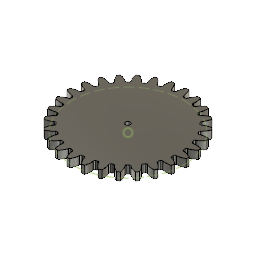
big_gear v6 (Autodesk Fusion 360 design; units mm, degrees)
description: Spur Gear; Module: 3.0; Num Teeth: 28; Pressure Angle: 20.0; Backlash: 0.00 mm
Autodesk Fusion 360 part; units mm, degrees
(part 1 of 4)
sketch "Sketch1" plane through (0, 0, 5) normal (0, 0, 1) x (-1, 0, 0)
  arc A0 (-25.3771, 2.9606) -> (-25.3996, 2.7606) centre (0, 0) ccw
  spline S0 degree 3 poles (-26.3672, 1.869) (-26.2575, 1.8719) (-26.149, 1.8929) (-25.9431, 1.9692) (-25.8472, 2.0241) (-25.6612, 2.1757) (-25.5772, 2.2768) (-25.4529, 2.5057) (-25.4137, 2.6311) (-25.3996, 2.7606) knots -0.143992 -0.143992 -0.143992 -0.143992 -0.11106 -0.11106 -0.078129 -0.078129 -0.039064 -0.039064 0 0 0 0
  spline S1 degree 3 poles (-29.9911, 0.731) (-29.3159, 1.0797) (-27.9521, 1.7065) (-26.5825, 1.8547) (-26.4748, 1.8661) (-26.3672, 1.869) knots -0.425485 -0.425485 -0.425485 -0.425485 -0.0445 -0.0445 -0.012227 -0.012227 -0.012227 -0.012227
  arc A1 (-29.9911, 0.731) -> (-29.9911, -0.731) centre (0, 0) ccw
  spline S2 degree 3 poles (-26.3672, -1.869) (-26.7354, -1.8592) (-27.3741, -1.7595) (-28.77, -1.3092) (-29.3991, -1.0367) (-29.9911, -0.731) knots -0.43899 -0.43899 -0.43899 -0.43899 -0.19989 -0.19989 0 0 0 0
  spline S3 degree 3 poles (-25.3996, -2.7606) (-25.4115, -2.6515) (-25.4412, -2.545) (-25.5341, -2.3461) (-25.5966, -2.255) (-25.7629, -2.0819) (-25.8706, -2.0065) (-26.1088, -1.9013) (-26.2371, -1.8725) (-26.3672, -1.869) knots -0.143992 -0.143992 -0.143992 -0.143992 -0.11106 -0.11106 -0.078129 -0.078129 -0.039064 -0.039064 0 0 0 0
  arc A2 (-25.3996, -2.7606) -> (-25.3771, -2.9606) centre (0, 0) ccw
  spline S4 degree 3 poles (-26.122, -4.0451) (-26.0157, -4.0179) (-25.9146, -3.9733) (-25.7309, -3.8531) (-25.6496, -3.7782) (-25.5019, -3.589) (-25.4426, -3.4717) (-25.3723, -3.221) (-25.362, -3.0899) (-25.3771, -2.9606) knots -0.143992 -0.143992 -0.143992 -0.143992 -0.11106 -0.11106 -0.078129 -0.078129 -0.039064 -0.039064 0 0 0 0
  spline S5 degree 3 poles (-29.4018, -5.961) (-28.8212, -5.4708) (-27.631, -4.5562) (-26.3288, -4.1069) (-26.2263, -4.0718) (-26.122, -4.0451) knots -0.425485 -0.425485 -0.425485 -0.425485 -0.0445 -0.0445 -0.012227 -0.012227 -0.012227 -0.012227
  arc A3 (-29.4018, -5.961) -> (-29.0765, -7.3863) centre (0, 0) ccw
  spline S6 degree 3 poles (-25.2903, -7.6894) (-25.6513, -7.7618) (-26.2963, -7.8067) (-27.7573, -7.6783) (-28.4313, -7.5527) (-29.0765, -7.3863) knots -0.43899 -0.43899 -0.43899 -0.43899 -0.19989 -0.19989 0 0 0 0
  spline S7 degree 3 poles (-24.1485, -8.3433) (-24.1844, -8.2396) (-24.237, -8.1424) (-24.3719, -7.9692) (-24.4531, -7.8942) (-24.6537, -7.7625) (-24.7755, -7.713) (-25.0311, -7.6634) (-25.1626, -7.6638) (-25.2903, -7.6894) knots -0.143992 -0.143992 -0.143992 -0.143992 -0.11106 -0.11106 -0.078129 -0.078129 -0.039064 -0.039064 0 0 0 0
  arc A4 (-24.1485, -8.3433) -> (-24.082, -8.5333) centre (0, 0) ccw
  spline S8 degree 3 poles (-24.567, -9.7564) (-24.4694, -9.7062) (-24.3807, -9.6402) (-24.2284, -9.4821) (-24.1657, -9.3911) (-24.0639, -9.1738) (-24.0322, -9.0462) (-24.0195, -8.7861) (-24.0386, -8.656) (-24.082, -8.5333) knots -0.143992 -0.143992 -0.143992 -0.143992 -0.11106 -0.11106 -0.078129 -0.078129 -0.039064 -0.039064 0 0 0 0
  spline S9 degree 3 poles (-27.3382, -12.3541) (-26.8812, -11.7469) (-25.9244, -10.5904) (-24.7548, -9.8627) (-24.6626, -9.8056) (-24.567, -9.7564) knots -0.425485 -0.425485 -0.425485 -0.425485 -0.0445 -0.0445 -0.012227 -0.012227 -0.012227 -0.012227
  arc A5 (-27.3382, -12.3541) -> (-26.7039, -13.6712) centre (0, 0) ccw
  spline S10 degree 3 poles (-22.9451, -13.1242) (-23.281, -13.2751) (-23.8998, -13.4625) (-25.3528, -13.6624) (-26.0379, -13.6899) (-26.7039, -13.6712) knots -0.43899 -0.43899 -0.43899 -0.43899 -0.19989 -0.19989 0 0 0 0
  spline S11 degree 3 poles (-21.6865, -13.5077) (-21.7445, -13.4145) (-21.8175, -13.3315) (-21.9875, -13.1926) (-22.0834, -13.1376) (-22.3083, -13.0538) (-22.438, -13.0327) (-22.6983, -13.0412) (-22.8263, -13.0709) (-22.9451, -13.1242) knots -0.143992 -0.143992 -0.143992 -0.143992 -0.11106 -0.11106 -0.078129 -0.078129 -0.039064 -0.039064 0 0 0 0
  arc A6 (-21.6865, -13.5077) -> (-21.5794, -13.6781) centre (0, 0) ccw
  spline S12 degree 3 poles (-21.78, -14.9785) (-21.6961, -14.9078) (-21.6243, -14.8237) (-21.5109, -14.6357) (-21.4701, -14.533) (-21.4192, -14.2985) (-21.4167, -14.167) (-21.4622, -13.9106) (-21.5097, -13.7881) (-21.5794, -13.6781) knots -0.143992 -0.143992 -0.143992 -0.143992 -0.11106 -0.11106 -0.078129 -0.078129 -0.039064 -0.039064 0 0 0 0
  spline S13 degree 3 poles (-23.9037, -18.1277) (-23.5933, -17.434) (-22.9178, -16.0936) (-21.9395, -15.1238) (-21.8623, -15.0477) (-21.78, -14.9785) knots -0.425485 -0.425485 -0.425485 -0.425485 -0.0445 -0.0445 -0.012227 -0.012227 -0.012227 -0.012227
  arc A7 (-23.9037, -18.1277) -> (-22.9922, -19.2706) centre (0, 0) ccw
  spline S14 degree 3 poles (-19.4494, -17.9009) (-19.7433, -18.1228) (-20.3049, -18.4432) (-21.677, -18.9614) (-22.3388, -19.1406) (-22.9922, -19.2706) knots -0.43899 -0.43899 -0.43899 -0.43899 -0.19989 -0.19989 0 0 0 0
  spline S15 degree 3 poles (-18.137, -17.9947) (-18.2143, -17.9168) (-18.304, -17.8521) (-18.5006, -17.7545) (-18.6063, -17.7222) (-18.8442, -17.6906) (-18.9754, -17.6988) (-19.2272, -17.7651) (-19.3455, -17.8225) (-19.4494, -17.9009) knots -0.143992 -0.143992 -0.143992 -0.143992 -0.11106 -0.11106 -0.078129 -0.078129 -0.039064 -0.039064 0 0 0 0
  arc A8 (-18.137, -17.9947) -> (-17.9947, -18.137) centre (0, 0) ccw
  spline S16 degree 3 poles (-17.9009, -19.4494) (-17.8348, -19.3618) (-17.7835, -19.2639) (-17.7149, -19.0554) (-17.6979, -18.9462) (-17.7005, -18.7062) (-17.7273, -18.5775) (-17.8286, -18.3376) (-17.9023, -18.2287) (-17.9947, -18.137) knots -0.143992 -0.143992 -0.143992 -0.143992 -0.11106 -0.11106 -0.078129 -0.078129 -0.039064 -0.039064 0 0 0 0
  spline S17 degree 3 poles (-19.2706, -22.9922) (-19.1223, -22.2469) (-18.762, -20.7898) (-18.024, -19.6266) (-17.9658, -19.5353) (-17.9009, -19.4494) knots -0.425485 -0.425485 -0.425485 -0.425485 -0.0445 -0.0445 -0.012227 -0.012227 -0.012227 -0.012227
  arc A9 (-19.2706, -22.9922) -> (-18.1277, -23.9037) centre (0, 0) ccw
  spline S18 degree 3 poles (-14.9785, -21.78) (-15.2156, -22.0617) (-15.6918, -22.499) (-16.9142, -23.3096) (-17.5195, -23.6315) (-18.1277, -23.9037) knots -0.43899 -0.43899 -0.43899 -0.43899 -0.19989 -0.19989 0 0 0 0
  spline S19 degree 3 poles (-13.6781, -21.5794) (-13.7708, -21.5207) (-13.8726, -21.4776) (-14.086, -21.4261) (-14.1962, -21.4182) (-14.4352, -21.4403) (-14.5613, -21.4775) (-14.7921, -21.5981) (-14.8946, -21.6804) (-14.9785, -21.78) knots -0.143992 -0.143992 -0.143992 -0.143992 -0.11106 -0.11106 -0.078129 -0.078129 -0.039064 -0.039064 0 0 0 0
  arc A10 (-13.6781, -21.5794) -> (-13.5077, -21.6865) centre (0, 0) ccw
  spline S20 degree 3 poles (-13.1242, -22.9451) (-13.0792, -22.845) (-13.051, -22.7381) (-13.0305, -22.5196) (-13.0383, -22.4093) (-13.0942, -22.1759) (-13.1489, -22.0564) (-13.3011, -21.8451) (-13.3972, -21.7553) (-13.5077, -21.6865) knots -0.143992 -0.143992 -0.143992 -0.143992 -0.11106 -0.11106 -0.078129 -0.078129 -0.039064 -0.039064 0 0 0 0
  spline S21 degree 3 poles (-13.6712, -26.7039) (-13.6925, -25.9443) (-13.6655, -24.4435) (-13.2048, -23.1453) (-13.1683, -23.0433) (-13.1242, -22.9451) knots -0.425485 -0.425485 -0.425485 -0.425485 -0.0445 -0.0445 -0.012227 -0.012227 -0.012227 -0.012227
  arc A11 (-13.6712, -26.7039) -> (-12.3541, -27.3382) centre (0, 0) ccw
  spline S22 degree 3 poles (-9.7564, -24.567) (-9.9249, -24.8944) (-10.2919, -25.4267) (-11.3032, -26.4889) (-11.8217, -26.9375) (-12.3541, -27.3382) knots -0.43899 -0.43899 -0.43899 -0.43899 -0.19989 -0.19989 0 0 0 0
  spline S23 degree 3 poles (-8.5333, -24.082) (-8.6367, -24.0454) (-8.7455, -24.026) (-8.9651, -24.0234) (-9.0743, -24.0401) (-9.3024, -24.1149) (-9.417, -24.1792) (-9.6152, -24.3482) (-9.6968, -24.4512) (-9.7564, -24.567) knots -0.143992 -0.143992 -0.143992 -0.143992 -0.11106 -0.11106 -0.078129 -0.078129 -0.039064 -0.039064 0 0 0 0
  arc A12 (-8.5333, -24.082) -> (-8.3433, -24.1485) centre (0, 0) ccw
  spline S24 degree 3 poles (-7.6894, -25.2903) (-7.6678, -25.1826) (-7.6641, -25.0722) (-7.6927, -24.8545) (-7.7249, -24.7488) (-7.8313, -24.5336) (-7.9112, -24.4293) (-8.1067, -24.2572) (-8.2203, -24.191) (-8.3433, -24.1485) knots -0.143992 -0.143992 -0.143992 -0.143992 -0.11106 -0.11106 -0.078129 -0.078129 -0.039064 -0.039064 0 0 0 0
  spline S25 degree 3 poles (-7.3863, -29.0765) (-7.576, -28.3406) (-7.8837, -26.8715) (-7.7234, -25.5033) (-7.7105, -25.3957) (-7.6894, -25.2903) knots -0.425485 -0.425485 -0.425485 -0.425485 -0.0445 -0.0445 -0.012227 -0.012227 -0.012227 -0.012227
  arc A13 (-7.3863, -29.0765) -> (-5.961, -29.4018) centre (0, 0) ccw
  spline S26 degree 3 poles (-4.0451, -26.122) (-4.1366, -26.4788) (-4.3759, -27.0793) (-5.1255, -28.34) (-5.5312, -28.8927) (-5.961, -29.4018) knots -0.43899 -0.43899 -0.43899 -0.43899 -0.19989 -0.19989 0 0 0 0
  spline S27 degree 3 poles (-2.9606, -25.3771) (-3.0696, -25.3644) (-3.18, -25.3697) (-3.3946, -25.416) (-3.4974, -25.4566) (-3.7031, -25.5802) (-3.8005, -25.6685) (-3.9561, -25.8773) (-4.0128, -25.9959) (-4.0451, -26.122) knots -0.143992 -0.143992 -0.143992 -0.143992 -0.11106 -0.11106 -0.078129 -0.078129 -0.039064 -0.039064 0 0 0 0
  arc A14 (-2.9606, -25.3771) -> (-2.7606, -25.3996) centre (0, 0) ccw
  spline S28 degree 3 poles (-1.869, -26.3672) (-1.8719, -26.2575) (-1.8929, -26.149) (-1.9692, -25.9431) (-2.0241, -25.8472) (-2.1757, -25.6612) (-2.2768, -25.5772) (-2.5057, -25.4529) (-2.6311, -25.4137) (-2.7606, -25.3996) knots -0.143992 -0.143992 -0.143992 -0.143992 -0.11106 -0.11106 -0.078129 -0.078129 -0.039064 -0.039064 0 0 0 0
  spline S29 degree 3 poles (-0.731, -29.9911) (-1.0797, -29.3159) (-1.7065, -27.9521) (-1.8547, -26.5825) (-1.8661, -26.4748) (-1.869, -26.3672) knots -0.425485 -0.425485 -0.425485 -0.425485 -0.0445 -0.0445 -0.012227 -0.012227 -0.012227 -0.012227
  arc A15 (-0.731, -29.9911) -> (0.731, -29.9911) centre (0, 0) ccw
  spline S30 degree 3 poles (1.869, -26.3672) (1.8592, -26.7354) (1.7595, -27.3741) (1.3092, -28.77) (1.0367, -29.3991) (0.731, -29.9911) knots -0.43899 -0.43899 -0.43899 -0.43899 -0.19989 -0.19989 0 0 0 0
  spline S31 degree 3 poles (2.7606, -25.3996) (2.6515, -25.4115) (2.545, -25.4412) (2.3461, -25.5341) (2.255, -25.5966) (2.0819, -25.7629) (2.0065, -25.8706) (1.9013, -26.1088) (1.8725, -26.2371) (1.869, -26.3672) knots -0.143992 -0.143992 -0.143992 -0.143992 -0.11106 -0.11106 -0.078129 -0.078129 -0.039064 -0.039064 0 0 0 0
  arc A16 (2.7606, -25.3996) -> (2.9606, -25.3771) centre (0, 0) ccw
  spline S32 degree 3 poles (4.0451, -26.122) (4.0179, -26.0157) (3.9733, -25.9146) (3.8531, -25.7309) (3.7782, -25.6496) (3.589, -25.5019) (3.4717, -25.4426) (3.221, -25.3723) (3.0899, -25.362) (2.9606, -25.3771) knots -0.143992 -0.143992 -0.143992 -0.143992 -0.11106 -0.11106 -0.078129 -0.078129 -0.039064 -0.039064 0 0 0 0
  spline S33 degree 3 poles (5.961, -29.4018) (5.4708, -28.8212) (4.5562, -27.631) (4.1069, -26.3288) (4.0718, -26.2263) (4.0451, -26.122) knots -0.425485 -0.425485 -0.425485 -0.425485 -0.0445 -0.0445 -0.012227 -0.012227 -0.012227 -0.012227
  arc A17 (5.961, -29.4018) -> (7.3863, -29.0765) centre (0, 0) ccw
  spline S34 degree 3 poles (7.6894, -25.2903) (7.7618, -25.6513) (7.8067, -26.2963) (7.6783, -27.7573) (7.5527, -28.4313) (7.3863, -29.0765) knots -0.43899 -0.43899 -0.43899 -0.43899 -0.19989 -0.19989 0 0 0 0
  spline S35 degree 3 poles (8.3433, -24.1485) (8.2396, -24.1844) (8.1424, -24.237) (7.9692, -24.3719) (7.8942, -24.4531) (7.7625, -24.6537) (7.713, -24.7755) (7.6634, -25.0311) (7.6638, -25.1626) (7.6894, -25.2903) knots -0.143992 -0.143992 -0.143992 -0.143992 -0.11106 -0.11106 -0.078129 -0.078129 -0.039064 -0.039064 0 0 0 0
  arc A18 (8.3433, -24.1485) -> (8.5333, -24.082) centre (0, 0) ccw
  spline S36 degree 3 poles (9.7564, -24.567) (9.7062, -24.4694) (9.6402, -24.3807) (9.4821, -24.2284) (9.3911, -24.1657) (9.1738, -24.0639) (9.0462, -24.0322) (8.7861, -24.0195) (8.656, -24.0386) (8.5333, -24.082) knots -0.143992 -0.143992 -0.143992 -0.143992 -0.11106 -0.11106 -0.078129 -0.078129 -0.039064 -0.039064 0 0 0 0
  spline S37 degree 3 poles (12.3541, -27.3382) (11.7469, -26.8812) (10.5904, -25.9244) (9.8627, -24.7548) (9.8056, -24.6626) (9.7564, -24.567) knots -0.425485 -0.425485 -0.425485 -0.425485 -0.0445 -0.0445 -0.012227 -0.012227 -0.012227 -0.012227
  arc A19 (12.3541, -27.3382) -> (13.6712, -26.7039) centre (0, 0) ccw
  spline S38 degree 3 poles (13.1242, -22.9451) (13.2751, -23.281) (13.4625, -23.8998) (13.6624, -25.3528) (13.6899, -26.0379) (13.6712, -26.7039) knots -0.43899 -0.43899 -0.43899 -0.43899 -0.19989 -0.19989 0 0 0 0
  spline S39 degree 3 poles (13.5077, -21.6865) (13.4145, -21.7445) (13.3315, -21.8175) (13.1926, -21.9875) (13.1376, -22.0834) (13.0538, -22.3083) (13.0327, -22.438) (13.0412, -22.6983) (13.0709, -22.8263) (13.1242, -22.9451) knots -0.143992 -0.143992 -0.143992 -0.143992 -0.11106 -0.11106 -0.078129 -0.078129 -0.039064 -0.039064 0 0 0 0
  arc A20 (13.5077, -21.6865) -> (13.6781, -21.5794) centre (0, 0) ccw
  spline S40 degree 3 poles (14.9785, -21.78) (14.9078, -21.6961) (14.8237, -21.6243) (14.6357, -21.5109) (14.533, -21.4701) (14.2985, -21.4192) (14.167, -21.4167) (13.9106, -21.4622) (13.7881, -21.5097) (13.6781, -21.5794) knots -0.143992 -0.143992 -0.143992 -0.143992 -0.11106 -0.11106 -0.078129 -0.078129 -0.039064 -0.039064 0 0 0 0
  spline S41 degree 3 poles (18.1277, -23.9037) (17.434, -23.5933) (16.0936, -22.9178) (15.1238, -21.9395) (15.0477, -21.8623) (14.9785, -21.78) knots -0.425485 -0.425485 -0.425485 -0.425485 -0.0445 -0.0445 -0.012227 -0.012227 -0.012227 -0.012227
  arc A21 (18.1277, -23.9037) -> (19.2706, -22.9922) centre (0, 0) ccw
  spline S42 degree 3 poles (17.9009, -19.4494) (18.1228, -19.7433) (18.4432, -20.3049) (18.9614, -21.677) (19.1406, -22.3388) (19.2706, -22.9922) knots -0.43899 -0.43899 -0.43899 -0.43899 -0.19989 -0.19989 0 0 0 0
  spline S43 degree 3 poles (17.9947, -18.137) (17.9168, -18.2143) (17.8521, -18.304) (17.7545, -18.5006) (17.7222, -18.6063) (17.6906, -18.8442) (17.6988, -18.9754) (17.7651, -19.2272) (17.8225, -19.3455) (17.9009, -19.4494) knots -0.143992 -0.143992 -0.143992 -0.143992 -0.11106 -0.11106 -0.078129 -0.078129 -0.039064 -0.039064 0 0 0 0
  arc A22 (17.9947, -18.137) -> (18.137, -17.9947) centre (0, 0) ccw
  spline S44 degree 3 poles (19.4494, -17.9009) (19.3618, -17.8348) (19.2639, -17.7835) (19.0554, -17.7149) (18.9462, -17.6979) (18.7062, -17.7005) (18.5775, -17.7273) (18.3376, -17.8286) (18.2287, -17.9023) (18.137, -17.9947) knots -0.143992 -0.143992 -0.143992 -0.143992 -0.11106 -0.11106 -0.078129 -0.078129 -0.039064 -0.039064 0 0 0 0
  spline S45 degree 3 poles (22.9922, -19.2706) (22.2469, -19.1223) (20.7898, -18.762) (19.6266, -18.024) (19.5353, -17.9658) (19.4494, -17.9009) knots -0.425485 -0.425485 -0.425485 -0.425485 -0.0445 -0.0445 -0.012227 -0.012227 -0.012227 -0.012227
  arc A23 (22.9922, -19.2706) -> (23.9037, -18.1277) centre (0, 0) ccw
  spline S46 degree 3 poles (21.78, -14.9785) (22.0617, -15.2156) (22.499, -15.6918) (23.3096, -16.9142) (23.6315, -17.5195) (23.9037, -18.1277) knots -0.43899 -0.43899 -0.43899 -0.43899 -0.19989 -0.19989 0 0 0 0
  spline S47 degree 3 poles (21.5794, -13.6781) (21.5207, -13.7708) (21.4776, -13.8726) (21.4261, -14.086) (21.4182, -14.1962) (21.4403, -14.4352) (21.4775, -14.5613) (21.5981, -14.7921) (21.6804, -14.8946) (21.78, -14.9785) knots -0.143992 -0.143992 -0.143992 -0.143992 -0.11106 -0.11106 -0.078129 -0.078129 -0.039064 -0.039064 0 0 0 0
  arc A24 (21.5794, -13.6781) -> (21.6865, -13.5077) centre (0, 0) ccw
  spline S48 degree 3 poles (22.9451, -13.1242) (22.845, -13.0792) (22.7381, -13.051) (22.5196, -13.0305) (22.4093, -13.0383) (22.1759, -13.0942) (22.0564, -13.1489) (21.8451, -13.3011) (21.7553, -13.3972) (21.6865, -13.5077) knots -0.143992 -0.143992 -0.143992 -0.143992 -0.11106 -0.11106 -0.078129 -0.078129 -0.039064 -0.039064 0 0 0 0
  spline S49 degree 3 poles (26.7039, -13.6712) (25.9443, -13.6925) (24.4435, -13.6655) (23.1453, -13.2048) (23.0433, -13.1683) (22.9451, -13.1242) knots -0.425485 -0.425485 -0.425485 -0.425485 -0.0445 -0.0445 -0.012227 -0.012227 -0.012227 -0.012227
  arc A25 (26.7039, -13.6712) -> (27.3382, -12.3541) centre (0, 0) ccw
  spline S50 degree 3 poles (24.567, -9.7564) (24.8944, -9.9249) (25.4267, -10.2919) (26.4889, -11.3032) (26.9375, -11.8217) (27.3382, -12.3541) knots -0.43899 -0.43899 -0.43899 -0.43899 -0.19989 -0.19989 0 0 0 0
  spline S51 degree 3 poles (24.082, -8.5333) (24.0454, -8.6367) (24.026, -8.7455) (24.0234, -8.9651) (24.0401, -9.0743) (24.1149, -9.3024) (24.1792, -9.417) (24.3482, -9.6152) (24.4512, -9.6968) (24.567, -9.7564) knots -0.143992 -0.143992 -0.143992 -0.143992 -0.11106 -0.11106 -0.078129 -0.078129 -0.039064 -0.039064 0 0 0 0
  arc A26 (24.082, -8.5333) -> (24.1485, -8.3433) centre (0, 0) ccw
  spline S52 degree 3 poles (25.2903, -7.6894) (25.1826, -7.6678) (25.0722, -7.6641) (24.8545, -7.6927) (24.7488, -7.7249) (24.5336, -7.8313) (24.4293, -7.9112) (24.2572, -8.1067) (24.191, -8.2203) (24.1485, -8.3433) knots -0.143992 -0.143992 -0.143992 -0.143992 -0.11106 -0.11106 -0.078129 -0.078129 -0.039064 -0.039064 0 0 0 0
  spline S53 degree 3 poles (29.0765, -7.3863) (28.3406, -7.576) (26.8715, -7.8837) (25.5033, -7.7234) (25.3957, -7.7105) (25.2903, -7.6894) knots -0.425485 -0.425485 -0.425485 -0.425485 -0.0445 -0.0445 -0.012227 -0.012227 -0.012227 -0.012227
  arc A27 (29.0765, -7.3863) -> (29.4018, -5.961) centre (0, 0) ccw
  spline S54 degree 3 poles (26.122, -4.0451) (26.4788, -4.1366) (27.0793, -4.3759) (28.34, -5.1255) (28.8927, -5.5312) (29.4018, -5.961) knots -0.43899 -0.43899 -0.43899 -0.43899 -0.19989 -0.19989 0 0 0 0
  spline S55 degree 3 poles (25.3771, -2.9606) (25.3644, -3.0696) (25.3697, -3.18) (25.416, -3.3946) (25.4566, -3.4974) (25.5802, -3.7031) (25.6685, -3.8005) (25.8773, -3.9561) (25.9959, -4.0128) (26.122, -4.0451) knots -0.143992 -0.143992 -0.143992 -0.143992 -0.11106 -0.11106 -0.078129 -0.078129 -0.039064 -0.039064 0 0 0 0
  arc A28 (25.3771, -2.9606) -> (25.3996, -2.7606) centre (0, 0) ccw
  spline S56 degree 3 poles (26.3672, -1.869) (26.2575, -1.8719) (26.149, -1.8929) (25.9431, -1.9692) (25.8472, -2.0241) (25.6612, -2.1757) (25.5772, -2.2768) (25.4529, -2.5057) (25.4137, -2.6311) (25.3996, -2.7606) knots -0.143992 -0.143992 -0.143992 -0.143992 -0.11106 -0.11106 -0.078129 -0.078129 -0.039064 -0.039064 0 0 0 0
  spline S57 degree 3 poles (29.9911, -0.731) (29.3159, -1.0797) (27.9521, -1.7065) (26.5825, -1.8547) (26.4748, -1.8661) (26.3672, -1.869) knots -0.425485 -0.425485 -0.425485 -0.425485 -0.0445 -0.0445 -0.012227 -0.012227 -0.012227 -0.012227
  arc A29 (29.9911, -0.731) -> (29.9911, 0.731) centre (0, 0) ccw
  spline S58 degree 3 poles (26.3672, 1.869) (26.7354, 1.8592) (27.3741, 1.7595) (28.77, 1.3092) (29.3991, 1.0367) (29.9911, 0.731) knots -0.43899 -0.43899 -0.43899 -0.43899 -0.19989 -0.19989 0 0 0 0
  spline S59 degree 3 poles (25.3996, 2.7606) (25.4115, 2.6515) (25.4412, 2.545) (25.5341, 2.3461) (25.5966, 2.255) (25.7629, 2.0819) (25.8706, 2.0065) (26.1088, 1.9013) (26.2371, 1.8725) (26.3672, 1.869) knots -0.143992 -0.143992 -0.143992 -0.143992 -0.11106 -0.11106 -0.078129 -0.078129 -0.039064 -0.039064 0 0 0 0
  arc A30 (25.3996, 2.7606) -> (25.3771, 2.9606) centre (0, 0) ccw
  spline S60 degree 3 poles (26.122, 4.0451) (26.0157, 4.0179) (25.9146, 3.9733) (25.7309, 3.8531) (25.6496, 3.7782) (25.5019, 3.589) (25.4426, 3.4717) (25.3723, 3.221) (25.362, 3.0899) (25.3771, 2.9606) knots -0.143992 -0.143992 -0.143992 -0.143992 -0.11106 -0.11106 -0.078129 -0.078129 -0.039064 -0.039064 0 0 0 0
  spline S61 degree 3 poles (29.4018, 5.961) (28.8212, 5.4708) (27.631, 4.5562) (26.3288, 4.1069) (26.2263, 4.0718) (26.122, 4.0451) knots -0.425485 -0.425485 -0.425485 -0.425485 -0.0445 -0.0445 -0.012227 -0.012227 -0.012227 -0.012227
  arc A31 (29.4018, 5.961) -> (29.0765, 7.3863) centre (0, 0) ccw
  spline S62 degree 3 poles (25.2903, 7.6894) (25.6513, 7.7618) (26.2963, 7.8067) (27.7573, 7.6783) (28.4313, 7.5527) (29.0765, 7.3863) knots -0.43899 -0.43899 -0.43899 -0.43899 -0.19989 -0.19989 0 0 0 0
  spline S63 degree 3 poles (24.1485, 8.3433) (24.1844, 8.2396) (24.237, 8.1424) (24.3719, 7.9692) (24.4531, 7.8942) (24.6537, 7.7625) (24.7755, 7.713) (25.0311, 7.6634) (25.1626, 7.6638) (25.2903, 7.6894) knots -0.143992 -0.143992 -0.143992 -0.143992 -0.11106 -0.11106 -0.078129 -0.078129 -0.039064 -0.039064 0 0 0 0
  arc A32 (24.1485, 8.3433) -> (24.082, 8.5333) centre (0, 0) ccw
  spline S64 degree 3 poles (24.567, 9.7564) (24.4694, 9.7062) (24.3807, 9.6402) (24.2284, 9.4821) (24.1657, 9.3911) (24.0639, 9.1738) (24.0322, 9.0462) (24.0195, 8.7861) (24.0386, 8.656) (24.082, 8.5333) knots -0.143992 -0.143992 -0.143992 -0.143992 -0.11106 -0.11106 -0.078129 -0.078129 -0.039064 -0.039064 0 0 0 0
  spline S65 degree 3 poles (27.3382, 12.3541) (26.8812, 11.7469) (25.9244, 10.5904) (24.7548, 9.8627) (24.6626, 9.8056) (24.567, 9.7564) knots -0.425485 -0.425485 -0.425485 -0.425485 -0.0445 -0.0445 -0.012227 -0.012227 -0.012227 -0.012227
  arc A33 (27.3382, 12.3541) -> (26.7039, 13.6712) centre (0, 0) ccw
  spline S66 degree 3 poles (22.9451, 13.1242) (23.281, 13.2751) (23.8998, 13.4625) (25.3528, 13.6624) (26.0379, 13.6899) (26.7039, 13.6712) knots -0.43899 -0.43899 -0.43899 -0.43899 -0.19989 -0.19989 0 0 0 0
  spline S67 degree 3 poles (21.6865, 13.5077) (21.7445, 13.4145) (21.8175, 13.3315) (21.9875, 13.1926) (22.0834, 13.1376) (22.3083, 13.0538) (22.438, 13.0327) (22.6983, 13.0412) (22.8263, 13.0709) (22.9451, 13.1242) knots -0.143992 -0.143992 -0.143992 -0.143992 -0.11106 -0.11106 -0.078129 -0.078129 -0.039064 -0.039064 0 0 0 0
  arc A34 (21.6865, 13.5077) -> (21.5794, 13.6781) centre (0, 0) ccw
  spline S68 degree 3 poles (21.78, 14.9785) (21.6961, 14.9078) (21.6243, 14.8237) (21.5109, 14.6357) (21.4701, 14.533) (21.4192, 14.2985) (21.4167, 14.167) (21.4622, 13.9106) (21.5097, 13.7881) (21.5794, 13.6781) knots -0.143992 -0.143992 -0.143992 -0.143992 -0.11106 -0.11106 -0.078129 -0.078129 -0.039064 -0.039064 0 0 0 0
  spline S69 degree 3 poles (23.9037, 18.1277) (23.5933, 17.434) (22.9178, 16.0936) (21.9395, 15.1238) (21.8623, 15.0477) (21.78, 14.9785) knots -0.425485 -0.425485 -0.425485 -0.425485 -0.0445 -0.0445 -0.012227 -0.012227 -0.012227 -0.012227
  arc A35 (23.9037, 18.1277) -> (22.9922, 19.2706) centre (0, 0) ccw
  spline S70 degree 3 poles (19.4494, 17.9009) (19.7433, 18.1228) (20.3049, 18.4432) (21.677, 18.9614) (22.3388, 19.1406) (22.9922, 19.2706) knots -0.43899 -0.43899 -0.43899 -0.43899 -0.19989 -0.19989 0 0 0 0
  spline S71 degree 3 poles (18.137, 17.9947) (18.2143, 17.9168) (18.304, 17.8521) (18.5006, 17.7545) (18.6063, 17.7222) (18.8442, 17.6906) (18.9754, 17.6988) (19.2272, 17.7651) (19.3455, 17.8225) (19.4494, 17.9009) knots -0.143992 -0.143992 -0.143992 -0.143992 -0.11106 -0.11106 -0.078129 -0.078129 -0.039064 -0.039064 0 0 0 0
  arc A36 (18.137, 17.9947) -> (17.9947, 18.137) centre (0, 0) ccw
  spline S72 degree 3 poles (17.9009, 19.4494) (17.8348, 19.3618) (17.7835, 19.2639) (17.7149, 19.0554) (17.6979, 18.9462) (17.7005, 18.7062) (17.7273, 18.5775) (17.8286, 18.3376) (17.9023, 18.2287) (17.9947, 18.137) knots -0.143992 -0.143992 -0.143992 -0.143992 -0.11106 -0.11106 -0.078129 -0.078129 -0.039064 -0.039064 0 0 0 0
  spline S73 degree 3 poles (19.2706, 22.9922) (19.1223, 22.2469) (18.762, 20.7898) (18.024, 19.6266) (17.9658, 19.5353) (17.9009, 19.4494) knots -0.425485 -0.425485 -0.425485 -0.425485 -0.0445 -0.0445 -0.012227 -0.012227 -0.012227 -0.012227
  arc A37 (19.2706, 22.9922) -> (18.1277, 23.9037) centre (0, 0) ccw
  spline S74 degree 3 poles (14.9785, 21.78) (15.2156, 22.0617) (15.6918, 22.499) (16.9142, 23.3096) (17.5195, 23.6315) (18.1277, 23.9037) knots -0.43899 -0.43899 -0.43899 -0.43899 -0.19989 -0.19989 0 0 0 0
  spline S75 degree 3 poles (13.6781, 21.5794) (13.7708, 21.5207) (13.8726, 21.4776) (14.086, 21.4261) (14.1962, 21.4182) (14.4352, 21.4403) (14.5613, 21.4775) (14.7921, 21.5981) (14.8946, 21.6804) (14.9785, 21.78) knots -0.143992 -0.143992 -0.143992 -0.143992 -0.11106 -0.11106 -0.078129 -0.078129 -0.039064 -0.039064 0 0 0 0
  arc A38 (13.6781, 21.5794) -> (13.5077, 21.6865) centre (0, 0) ccw
  spline S76 degree 3 poles (13.1242, 22.9451) (13.0792, 22.845) (13.051, 22.7381) (13.0305, 22.5196) (13.0383, 22.4093) (13.0942, 22.1759) (13.1489, 22.0564) (13.3011, 21.8451) (13.3972, 21.7553) (13.5077, 21.6865) knots -0.143992 -0.143992 -0.143992 -0.143992 -0.11106 -0.11106 -0.078129 -0.078129 -0.039064 -0.039064 0 0 0 0
  spline S77 degree 3 poles (13.6712, 26.7039) (13.6925, 25.9443) (13.6655, 24.4435) (13.2048, 23.1453) (13.1683, 23.0433) (13.1242, 22.9451) knots -0.425485 -0.425485 -0.425485 -0.425485 -0.0445 -0.0445 -0.012227 -0.012227 -0.012227 -0.012227
  arc A39 (13.6712, 26.7039) -> (12.3541, 27.3382) centre (0, 0) ccw
  spline S78 degree 3 poles (9.7564, 24.567) (9.9249, 24.8944) (10.2919, 25.4267) (11.3032, 26.4889) (11.8217, 26.9375) (12.3541, 27.3382) knots -0.43899 -0.43899 -0.43899 -0.43899 -0.19989 -0.19989 0 0 0 0
  spline S79 degree 3 poles (8.5333, 24.082) (8.6367, 24.0454) (8.7455, 24.026) (8.9651, 24.0234) (9.0743, 24.0401) (9.3024, 24.1149) (9.417, 24.1792) (9.6152, 24.3482) (9.6968, 24.4512) (9.7564, 24.567) knots -0.143992 -0.143992 -0.143992 -0.143992 -0.11106 -0.11106 -0.078129 -0.078129 -0.039064 -0.039064 0 0 0 0
  arc A40 (8.5333, 24.082) -> (8.3433, 24.1485) centre (0, 0) ccw
  spline S80 degree 3 poles (7.6894, 25.2903) (7.6678, 25.1826) (7.6641, 25.0722) (7.6927, 24.8545) (7.7249, 24.7488) (7.8313, 24.5336) (7.9112, 24.4293) (8.1067, 24.2572) (8.2203, 24.191) (8.3433, 24.1485) knots -0.143992 -0.143992 -0.143992 -0.143992 -0.11106 -0.11106 -0.078129 -0.078129 -0.039064 -0.039064 0 0 0 0
  spline S81 degree 3 poles (7.3863, 29.0765) (7.576, 28.3406) (7.8837, 26.8715) (7.7234, 25.5033) (7.7105, 25.3957) (7.6894, 25.2903) knots -0.425485 -0.425485 -0.425485 -0.425485 -0.0445 -0.0445 -0.012227 -0.012227 -0.012227 -0.012227
  arc A41 (7.3863, 29.0765) -> (5.961, 29.4018) centre (0, 0) ccw
  spline S82 degree 3 poles (4.0451, 26.122) (4.1366, 26.4788) (4.3759, 27.0793) (5.1255, 28.34) (5.5312, 28.8927) (5.961, 29.4018) knots -0.43899 -0.43899 -0.43899 -0.43899 -0.19989 -0.19989 0 0 0 0
  spline S83 degree 3 poles (2.9606, 25.3771) (3.0696, 25.3644) (3.18, 25.3697) (3.3946, 25.416) (3.4974, 25.4566) (3.7031, 25.5802) (3.8005, 25.6685) (3.9561, 25.8773) (4.0128, 25.9959) (4.0451, 26.122) knots -0.143992 -0.143992 -0.143992 -0.143992 -0.11106 -0.11106 -0.078129 -0.078129 -0.039064 -0.039064 0 0 0 0
  arc A42 (2.9606, 25.3771) -> (2.7606, 25.3996) centre (0, 0) ccw
  spline S84 degree 3 poles (1.869, 26.3672) (1.8719, 26.2575) (1.8929, 26.149) (1.9692, 25.9431) (2.0241, 25.8472) (2.1757, 25.6612) (2.2768, 25.5772) (2.5057, 25.4529) (2.6311, 25.4137) (2.7606, 25.3996) knots -0.143992 -0.143992 -0.143992 -0.143992 -0.11106 -0.11106 -0.078129 -0.078129 -0.039064 -0.039064 0 0 0 0
  spline S85 degree 3 poles (0.731, 29.9911) (1.0797, 29.3159) (1.7065, 27.9521) (1.8547, 26.5825) (1.8661, 26.4748) (1.869, 26.3672) knots -0.425485 -0.425485 -0.425485 -0.425485 -0.0445 -0.0445 -0.012227 -0.012227 -0.012227 -0.012227
  arc A43 (0.731, 29.9911) -> (-0.731, 29.9911) centre (0, 0) ccw
  spline S86 degree 3 poles (-1.869, 26.3672) (-1.8592, 26.7354) (-1.7595, 27.3741) (-1.3092, 28.77) (-1.0367, 29.3991) (-0.731, 29.9911) knots -0.43899 -0.43899 -0.43899 -0.43899 -0.19989 -0.19989 0 0 0 0
  spline S87 degree 3 poles (-2.7606, 25.3996) (-2.6515, 25.4115) (-2.545, 25.4412) (-2.3461, 25.5341) (-2.255, 25.5966) (-2.0819, 25.7629) (-2.0065, 25.8706) (-1.9013, 26.1088) (-1.8725, 26.2371) (-1.869, 26.3672) knots -0.143992 -0.143992 -0.143992 -0.143992 -0.11106 -0.11106 -0.078129 -0.078129 -0.039064 -0.039064 0 0 0 0
  arc A44 (-2.7606, 25.3996) -> (-2.9606, 25.3771) centre (0, 0) ccw
  spline S88 degree 3 poles (-4.0451, 26.122) (-4.0179, 26.0157) (-3.9733, 25.9146) (-3.8531, 25.7309) (-3.7782, 25.6496) (-3.589, 25.5019) (-3.4717, 25.4426) (-3.221, 25.3723) (-3.0899, 25.362) (-2.9606, 25.3771) knots -0.143992 -0.143992 -0.143992 -0.143992 -0.11106 -0.11106 -0.078129 -0.078129 -0.039064 -0.039064 0 0 0 0
  spline S89 degree 3 poles (-5.961, 29.4018) (-5.4708, 28.8212) (-4.5562, 27.631) (-4.1069, 26.3288) (-4.0718, 26.2263) (-4.0451, 26.122) knots -0.425485 -0.425485 -0.425485 -0.425485 -0.0445 -0.0445 -0.012227 -0.012227 -0.012227 -0.012227
  arc A45 (-5.961, 29.4018) -> (-7.3863, 29.0765) centre (0, 0) ccw
  spline S90 degree 3 poles (-7.6894, 25.2903) (-7.7618, 25.6513) (-7.8067, 26.2963) (-7.6783, 27.7573) (-7.5527, 28.4313) (-7.3863, 29.0765) knots -0.43899 -0.43899 -0.43899 -0.43899 -0.19989 -0.19989 0 0 0 0
  spline S91 degree 3 poles (-8.3433, 24.1485) (-8.2396, 24.1844) (-8.1424, 24.237) (-7.9692, 24.3719) (-7.8942, 24.4531) (-7.7625, 24.6537) (-7.713, 24.7755) (-7.6634, 25.0311) (-7.6638, 25.1626) (-7.6894, 25.2903) knots -0.143992 -0.143992 -0.143992 -0.143992 -0.11106 -0.11106 -0.078129 -0.078129 -0.039064 -0.039064 0 0 0 0
  arc A46 (-8.3433, 24.1485) -> (-8.5333, 24.082) centre (0, 0) ccw
  spline S92 degree 3 poles (-9.7564, 24.567) (-9.7062, 24.4694) (-9.6402, 24.3807) (-9.4821, 24.2284) (-9.3911, 24.1657) (-9.1738, 24.0639) (-9.0462, 24.0322) (-8.7861, 24.0195) (-8.656, 24.0386) (-8.5333, 24.082) knots -0.143992 -0.143992 -0.143992 -0.143992 -0.11106 -0.11106 -0.078129 -0.078129 -0.039064 -0.039064 0 0 0 0
  spline S93 degree 3 poles (-12.3541, 27.3382) (-11.7469, 26.8812) (-10.5904, 25.9244) (-9.8627, 24.7548) (-9.8056, 24.6626) (-9.7564, 24.567) knots -0.425485 -0.425485 -0.425485 -0.425485 -0.0445 -0.0445 -0.012227 -0.012227 -0.012227 -0.012227
  arc A47 (-12.3541, 27.3382) -> (-13.6712, 26.7039) centre (0, 0) ccw
  spline S94 degree 3 poles (-13.1242, 22.9451) (-13.2751, 23.281) (-13.4625, 23.8998) (-13.6624, 25.3528) (-13.6899, 26.0379) (-13.6712, 26.7039) knots -0.43899 -0.43899 -0.43899 -0.43899 -0.19989 -0.19989 0 0 0 0
  spline S95 degree 3 poles (-13.5077, 21.6865) (-13.4145, 21.7445) (-13.3315, 21.8175) (-13.1926, 21.9875) (-13.1376, 22.0834) (-13.0538, 22.3083) (-13.0327, 22.438) (-13.0412, 22.6983) (-13.0709, 22.8263) (-13.1242, 22.9451) knots -0.143992 -0.143992 -0.143992 -0.143992 -0.11106 -0.11106 -0.078129 -0.078129 -0.039064 -0.039064 0 0 0 0
  arc A48 (-13.5077, 21.6865) -> (-13.6781, 21.5794) centre (0, 0) ccw
  spline S96 degree 3 poles (-14.9785, 21.78) (-14.9078, 21.6961) (-14.8237, 21.6243) (-14.6357, 21.5109) (-14.533, 21.4701) (-14.2985, 21.4192) (-14.167, 21.4167) (-13.9106, 21.4622) (-13.7881, 21.5097) (-13.6781, 21.5794) knots -0.143992 -0.143992 -0.143992 -0.143992 -0.11106 -0.11106 -0.078129 -0.078129 -0.039064 -0.039064 0 0 0 0
  spline S97 degree 3 poles (-18.1277, 23.9037) (-17.434, 23.5933) (-16.0936, 22.9178) (-15.1238, 21.9395) (-15.0477, 21.8623) (-14.9785, 21.78) knots -0.425485 -0.425485 -0.425485 -0.425485 -0.0445 -0.0445 -0.012227 -0.012227 -0.012227 -0.012227
  arc A49 (-18.1277, 23.9037) -> (-19.2706, 22.9922) centre (0, 0) ccw
  spline S98 degree 3 poles (-17.9009, 19.4494) (-18.1228, 19.7433) (-18.4432, 20.3049) (-18.9614, 21.677) (-19.1406, 22.3388) (-19.2706, 22.9922) knots -0.43899 -0.43899 -0.43899 -0.43899 -0.19989 -0.19989 0 0 0 0
  spline S99 degree 3 poles (-17.9947, 18.137) (-17.9168, 18.2143) (-17.8521, 18.304) (-17.7545, 18.5006) (-17.7222, 18.6063) (-17.6906, 18.8442) (-17.6988, 18.9754) (-17.7651, 19.2272) (-17.8225, 19.3455) (-17.9009, 19.4494) knots -0.143992 -0.143992 -0.143992 -0.143992 -0.11106 -0.11106 -0.078129 -0.078129 -0.039064 -0.039064 0 0 0 0
  arc A50 (-17.9947, 18.137) -> (-18.137, 17.9947) centre (0, 0) ccw
  spline S100 degree 3 poles (-19.4494, 17.9009) (-19.3618, 17.8348) (-19.2639, 17.7835) (-19.0554, 17.7149) (-18.9462, 17.6979) (-18.7062, 17.7005) (-18.5775, 17.7273) (-18.3376, 17.8286) (-18.2287, 17.9023) (-18.137, 17.9947) knots -0.143992 -0.143992 -0.143992 -0.143992 -0.11106 -0.11106 -0.078129 -0.078129 -0.039064 -0.039064 0 0 0 0
  spline S101 degree 3 poles (-22.9922, 19.2706) (-22.2469, 19.1223) (-20.7898, 18.762) (-19.6266, 18.024) (-19.5353, 17.9658) (-19.4494, 17.9009) knots -0.425485 -0.425485 -0.425485 -0.425485 -0.0445 -0.0445 -0.012227 -0.012227 -0.012227 -0.012227
  arc A51 (-22.9922, 19.2706) -> (-23.9037, 18.1277) centre (0, 0) ccw
  spline S102 degree 3 poles (-21.78, 14.9785) (-22.0617, 15.2156) (-22.499, 15.6918) (-23.3096, 16.9142) (-23.6315, 17.5195) (-23.9037, 18.1277) knots -0.43899 -0.43899 -0.43899 -0.43899 -0.19989 -0.19989 0 0 0 0
  spline S103 degree 3 poles (-21.5794, 13.6781) (-21.5207, 13.7708) (-21.4776, 13.8726) (-21.4261, 14.086) (-21.4182, 14.1962) (-21.4403, 14.4352) (-21.4775, 14.5613) (-21.5981, 14.7921) (-21.6804, 14.8946) (-21.78, 14.9785) knots -0.143992 -0.143992 -0.143992 -0.143992 -0.11106 -0.11106 -0.078129 -0.078129 -0.039064 -0.039064 0 0 0 0
  arc A52 (-21.5794, 13.6781) -> (-21.6865, 13.5077) centre (0, 0) ccw
  spline S104 degree 3 poles (-22.9451, 13.1242) (-22.845, 13.0792) (-22.7381, 13.051) (-22.5196, 13.0305) (-22.4093, 13.0383) (-22.1759, 13.0942) (-22.0564, 13.1489) (-21.8451, 13.3011) (-21.7553, 13.3972) (-21.6865, 13.5077) knots -0.143992 -0.143992 -0.143992 -0.143992 -0.11106 -0.11106 -0.078129 -0.078129 -0.039064 -0.039064 0 0 0 0
  spline S105 degree 3 poles (-26.7039, 13.6712) (-25.9443, 13.6925) (-24.4435, 13.6655) (-23.1453, 13.2048) (-23.0433, 13.1683) (-22.9451, 13.1242) knots -0.425485 -0.425485 -0.425485 -0.425485 -0.0445 -0.0445 -0.012227 -0.012227 -0.012227 -0.012227
  arc A53 (-26.7039, 13.6712) -> (-27.3382, 12.3541) centre (0, 0) ccw
  spline S106 degree 3 poles (-24.567, 9.7564) (-24.8944, 9.9249) (-25.4267, 10.2919) (-26.4889, 11.3032) (-26.9375, 11.8217) (-27.3382, 12.3541) knots -0.43899 -0.43899 -0.43899 -0.43899 -0.19989 -0.19989 0 0 0 0
  spline S107 degree 3 poles (-24.082, 8.5333) (-24.0454, 8.6367) (-24.026, 8.7455) (-24.0234, 8.9651) (-24.0401, 9.0743) (-24.1149, 9.3024) (-24.1792, 9.417) (-24.3482, 9.6152) (-24.4512, 9.6968) (-24.567, 9.7564) knots -0.143992 -0.143992 -0.143992 -0.143992 -0.11106 -0.11106 -0.078129 -0.078129 -0.039064 -0.039064 0 0 0 0
  arc A54 (-24.082, 8.5333) -> (-24.1485, 8.3433) centre (0, 0) ccw
  spline S108 degree 3 poles (-25.2903, 7.6894) (-25.1826, 7.6678) (-25.0722, 7.6641) (-24.8545, 7.6927) (-24.7488, 7.7249) (-24.5336, 7.8313) (-24.4293, 7.9112) (-24.2572, 8.1067) (-24.191, 8.2203) (-24.1485, 8.3433) knots -0.143992 -0.143992 -0.143992 -0.143992 -0.11106 -0.11106 -0.078129 -0.078129 -0.039064 -0.039064 0 0 0 0
  spline S109 degree 3 poles (-29.0765, 7.3863) (-28.3406, 7.576) (-26.8715, 7.8837) (-25.5033, 7.7234) (-25.3957, 7.7105) (-25.2903, 7.6894) knots -0.425485 -0.425485 -0.425485 -0.425485 -0.0445 -0.0445 -0.012227 -0.012227 -0.012227 -0.012227
  arc A55 (-29.0765, 7.3863) -> (-29.4018, 5.961) centre (0, 0) ccw
  spline S110 degree 3 poles (-26.122, 4.0451) (-26.4788, 4.1366) (-27.0793, 4.3759) (-28.34, 5.1255) (-28.8927, 5.5312) (-29.4018, 5.961) knots -0.43899 -0.43899 -0.43899 -0.43899 -0.19989 -0.19989 0 0 0 0
  spline S111 degree 3 poles (-25.3771, 2.9606) (-25.3644, 3.0696) (-25.3697, 3.18) (-25.416, 3.3946) (-25.4566, 3.4974) (-25.5802, 3.7031) (-25.6685, 3.8005) (-25.8773, 3.9561) (-25.9959, 4.0128) (-26.122, 4.0451) knots -0.143992 -0.143992 -0.143992 -0.143992 -0.11106 -0.11106 -0.078129 -0.078129 -0.039064 -0.039064 0 0 0 0
  circle A56 centre (0, 0) radius 1.75
  line L0 (0, 0) -> (0, -23.5492)
  circle A57 centre (0, 0) radius 23.5492
  circle A58 centre (0, 0) radius 25.5492
  circle A59 centre (0, 0) radius 9
  circle A60 centre (0, 0) radius 11
  line L1 (1, -24.082) -> (-1, -24.082)
  line L2 (-1, -24.082) -> (-1, -10)
  line L3 (-1, -10) -> (1, -10)
  line L4 (1, -10) -> (1, -24.082)
  line L5 (9.1603, -4.134) -> (21.3557, -11.175)
  line L6 (20.3557, -12.907) -> (8.1603, -5.866)
  line L7 (8.1603, 5.866) -> (20.3557, 12.907)
  line L8 (21.3557, 11.175) -> (9.1603, 4.134)
  line L9 (-1, 10) -> (-1, 24.082)
  line L10 (1, 24.082) -> (1, 10)
  line L11 (-9.1603, 4.134) -> (-21.3557, 11.175)
  line L12 (-20.3557, 12.907) -> (-8.1603, 5.866)
  line L13 (-8.1603, -5.866) -> (-20.3557, -12.907)
  line L14 (-21.3557, -11.175) -> (-9.1603, -4.134)
  dimension "d23" = 2
  dimension "d24" = 18
  dimension "d25" = 2
  dimension "d26" = 1
  dimension "d27" = 1
  dimension "d29" = 360
  constraint coincident A0.centre A1.centre
  constraint vertical L0
  constraint concentric A0 A57
  constraint coincident L0.end A57
  constraint concentric A0 A58
  constraint coincident S31.start A58
  constraint concentric A57 A60
  constraint horizontal L1
  constraint vertical L2
  constraint horizontal L3
  constraint vertical L4
  measures "d23" distance of A57 A58
  measures "d24" diameter of A59
  measures "d25" distance of A59 A60
  measures "d26" distance of L0 L4
  measures "d27" distance of L0 L2
sketch "Sketch1 (2)" plane through (0, 0, 0) normal (0, 0, 1) x (1, 0, 0) in component "Spur Gear (28 teeth)"
  circle A0 centre (0, 0) radius 38.3492
  circle A1 centre (0, 0) radius 1.5
extrude "Extrude1" add sketch "Sketch1 (2)" along normal blind 5 in component "Spur Gear (28 teeth)"
sketch "Sketch2" plane through (0, 0, 0) normal (0, 0, 1) x (1, 0, 0) in component "Spur Gear (28 teeth)"
  spline S0 degree 5 poles (39.3676, -2.8) (39.3839, -2.8011) (39.4163, -2.803) (39.4649, -2.8047) (39.5299, -2.8047) (39.6111, -2.8017) (39.6923, -2.7966) (39.7736, -2.79) (39.855, -2.7828) (39.9363, -2.775) (40.0176, -2.7667) (40.099, -2.7577) (40.1803, -2.7478) (40.2616, -2.7369) (40.343, -2.7249) (40.4243, -2.7119) (40.5056, -2.6981) (40.5868, -2.6836) (40.6681, -2.6685) (40.7493, -2.6528) (40.8305, -2.6365) (40.9117, -2.6196) (40.9928, -2.6021) (41.074, -2.5839) (41.1551, -2.5651) (41.2361, -2.5457) (41.3171, -2.5256) (41.3981, -2.505) (41.4791, -2.4839) (41.56, -2.4622) (41.6408, -2.44) (41.7216, -2.4173) (41.8024, -2.3941) (41.8832, -2.3703) (41.9638, -2.346) (42.0445, -2.3213) (42.1251, -2.296) (42.2056, -2.2702) (42.2861, -2.244) (42.3666, -2.2173) (42.447, -2.1901) (42.5273, -2.1624) (42.6076, -2.1343) (42.6878, -2.1058) (42.768, -2.0768) (42.8481, -2.0473) (42.9282, -2.0174) (43.0082, -1.9871) (43.0881, -1.9563) (43.168, -1.9251) (43.2479, -1.8935) (43.3276, -1.8614) (43.4073, -1.829) (43.4869, -1.7961) (43.5665, -1.7628) (43.646, -1.7291) (43.7254, -1.695) (43.8048, -1.6605) (43.8841, -1.6256) (43.9633, -1.5903) (44.0425, -1.5546) (44.1216, -1.5185) (44.2006, -1.482) (44.2795, -1.4452) (44.3584, -1.4079) (44.4372, -1.3703) (44.5159, -1.3323) (44.5946, -1.2939) (44.6732, -1.2552) (44.7516, -1.2161) (44.8301, -1.1766) (44.8927, -1.1447) (44.9397, -1.1206) (44.971, -1.1045) (44.9866, -1.0964) knots 0 0 0 0 0 0 0.01428571 0.02857143 0.04285714 0.05714286 0.07142857 0.08571429 0.1 0.11428571 0.12857143 0.14285714 0.15714286 0.17142857 0.18571429 0.2 0.21428571 0.22857143 0.24285714 0.25714286 0.27142857 0.28571429 0.3 0.31428571 0.32857143 0.34285714 0.35714286 0.37142857 0.38571429 0.4 0.41428571 0.42857143 0.44285714 0.45714286 0.47142857 0.48571429 0.5 0.51428571 0.52857143 0.54285714 0.55714286 0.57142857 0.58571429 0.6 0.61428571 0.62857143 0.64285714 0.65714286 0.67142857 0.68571429 0.7 0.71428571 0.72857143 0.74285714 0.75714286 0.77142857 0.78571429 0.8 0.81428571 0.82857143 0.84285714 0.85714286 0.87142857 0.88571429 0.9 0.91428571 0.92857143 0.94285714 0.95714286 0.97142857 0.98571429 1 1 1 1 1 1
  spline S1 degree 5 poles (39.3676, 2.8) (39.3839, 2.8011) (39.4163, 2.803) (39.4649, 2.8047) (39.5299, 2.8047) (39.6111, 2.8017) (39.6923, 2.7966) (39.7736, 2.79) (39.855, 2.7828) (39.9363, 2.775) (40.0176, 2.7667) (40.099, 2.7577) (40.1803, 2.7478) (40.2616, 2.7369) (40.343, 2.7249) (40.4243, 2.7119) (40.5056, 2.6981) (40.5868, 2.6836) (40.6681, 2.6685) (40.7493, 2.6528) (40.8305, 2.6365) (40.9117, 2.6196) (40.9928, 2.6021) (41.074, 2.5839) (41.1551, 2.5651) (41.2361, 2.5457) (41.3171, 2.5256) (41.3981, 2.505) (41.4791, 2.4839) (41.56, 2.4622) (41.6408, 2.44) (41.7216, 2.4173) (41.8024, 2.3941) (41.8832, 2.3703) (41.9638, 2.346) (42.0445, 2.3213) (42.1251, 2.296) (42.2056, 2.2702) (42.2861, 2.244) (42.3666, 2.2173) (42.447, 2.1901) (42.5273, 2.1624) (42.6076, 2.1343) (42.6878, 2.1058) (42.768, 2.0768) (42.8481, 2.0473) (42.9282, 2.0174) (43.0082, 1.9871) (43.0881, 1.9563) (43.168, 1.9251) (43.2479, 1.8935) (43.3276, 1.8614) (43.4073, 1.829) (43.4869, 1.7961) (43.5665, 1.7628) (43.646, 1.7291) (43.7254, 1.695) (43.8048, 1.6605) (43.8841, 1.6256) (43.9633, 1.5903) (44.0425, 1.5546) (44.1216, 1.5185) (44.2006, 1.482) (44.2795, 1.4452) (44.3584, 1.4079) (44.4372, 1.3703) (44.5159, 1.3323) (44.5946, 1.2939) (44.6732, 1.2552) (44.7516, 1.2161) (44.8301, 1.1766) (44.8927, 1.1447) (44.9397, 1.1206) (44.971, 1.1045) (44.9866, 1.0964) knots 0 0 0 0 0 0 0.01428571 0.02857143 0.04285714 0.05714286 0.07142857 0.08571429 0.1 0.11428571 0.12857143 0.14285714 0.15714286 0.17142857 0.18571429 0.2 0.21428571 0.22857143 0.24285714 0.25714286 0.27142857 0.28571429 0.3 0.31428571 0.32857143 0.34285714 0.35714286 0.37142857 0.38571429 0.4 0.41428571 0.42857143 0.44285714 0.45714286 0.47142857 0.48571429 0.5 0.51428571 0.52857143 0.54285714 0.55714286 0.57142857 0.58571429 0.6 0.61428571 0.62857143 0.64285714 0.65714286 0.67142857 0.68571429 0.7 0.71428571 0.72857143 0.74285714 0.75714286 0.77142857 0.78571429 0.8 0.81428571 0.82857143 0.84285714 0.85714286 0.87142857 0.88571429 0.9 0.91428571 0.92857143 0.94285714 0.95714286 0.97142857 0.98571429 1 1 1 1 1 1
  arc A0 (44.9866, -1.0964) -> (44.9866, 1.0964) centre (0, 0) ccw
  line L0 (38.2426, -2.7207) -> (39.3676, -2.8)
  line L1 (38.2426, 2.7207) -> (39.3676, 2.8)
  line L2 (38.2426, -2.7207) -> (38.2426, 2.7207)
  point P0 (39.7645, -2.7906)
  point P1 (40.1635, -2.7497)
  point P2 (40.5638, -2.6876)
  point P3 (40.965, -2.608)
  point P4 (41.3669, -2.5129)
  point P5 (41.7692, -2.4036)
  point P6 (42.1719, -2.2809)
  point P7 (42.5747, -2.1458)
  point P8 (42.9775, -1.9987)
  point P9 (43.3802, -1.84)
  point P10 (43.7825, -1.6701)
  point P11 (44.1845, -1.4894)
  point P12 (44.5859, -1.2981)
  point P13 (39.7645, 2.7906)
  point P14 (40.1635, 2.7497)
  point P15 (40.5638, 2.6876)
  point P16 (40.965, 2.608)
  point P17 (41.3669, 2.5129)
  point P18 (41.7692, 2.4036)
  point P19 (42.1719, 2.2809)
  point P20 (42.5747, 2.1458)
  point P21 (42.9775, 1.9987)
  point P22 (43.3802, 1.84)
  point P23 (43.7825, 1.6701)
  point P24 (44.1845, 1.4894)
  point P25 (44.5859, 1.2981)
extrude "Extrude2" add sketch "Sketch2" along normal blind 5 in component "Spur Gear (28 teeth)"
fillet "Fillet1" radius 1 2 edges at (38.2525, -2.7214, 2.5) (38.2525, 2.7214, 2.5) in component "Spur Gear (28 teeth)"
pattern_circular "C-Pattern1" count 28 over 360 about axis through (0, 0, 0) along (0, 0, 1) of "Extrude2", "Fillet1" in component "Spur Gear (28 teeth)"
sketch "Sketch3" plane through (0, 0, 0) normal (0, 0, 1) x (1, 0, 0) in component "Spur Gear (28 teeth)"
  circle A0 centre (0, 0) radius 42 construction
extrude "Extrude3" add 1 faces at (0.0413, -25.9457, 5) along direction (0, 0, 1) blind 1 in component "Spur Gear (28 teeth)"